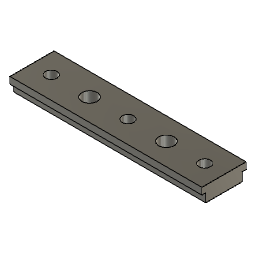
Alu_M6_M8_T-Track_Sliding_nut_T_100mm_holes_int (Autodesk Fusion 360 design; units mm, degrees)
Autodesk Fusion 360 part; units mm, degrees
sketch "Sketch1" plane through (0, 0, 0) normal (1, 0, 0) x (0, 1, 0)
  line L0 (0, 0) -> (9.5, 0)
  line L1 (0, 0) -> (0, 8) construction
  line L2 (0, 8) -> (11.5, 8)
  line L3 (11.5, 8) -> (11.5, 4.5)
  line L4 (11.5, 4.5) -> (9.5, 4.5)
  line L5 (9.5, 4.5) -> (9.5, 0)
  line L6 (-9.5, 4.5) -> (-9.5, 0)
  line L7 (-11.5, 8) -> (-11.5, 4.5)
  line L8 (0, 0) -> (-9.5, 0)
  line L9 (0, 8) -> (-11.5, 8)
  line L10 (-11.5, 4.5) -> (-9.5, 4.5)
  dimension "d1" = 9.5
  dimension "d2" = 8
  dimension "d3" = 11.5
  dimension "d4" = 3.5
  constraint coincident L0.start L1.start
  constraint horizontal L0
  constraint perpendicular L0 L1
  constraint perpendicular L1 L2
  constraint perpendicular L2 L3
  constraint perpendicular L3 L4
  constraint perpendicular L0 L5
  constraint symmetric L0.start L1 L8.start
  constraint symmetric L0.end L1 L6.end
  constraint symmetric L2.start L1 L9.start
  constraint symmetric L1 L2.end L7.start
  constraint symmetric L1 L3.end L7.end
  constraint symmetric L1 L4.end L6.start
  measures "d1" distance of L0.start L0.end
  measures "d2" distance of L0.start L1.end
  measures "d3" distance of L1.end L2.end
  measures "d4" distance of L2.end L3.end
extrude "Extrude1" add sketch "Sketch1" along normal mid plane 100
sketch "Sketch2" plane through (0, 0, 8) normal (0, 0, 1) x (-1, 0, 0)
  line L0 (50, 11.5) -> (-50, 11.5)
  line L1 (-50, 11.5) -> (-50, -11.5)
  line L2 (-50, -11.5) -> (50, -11.5)
  line L3 (50, -11.5) -> (50, 11.5)
  line L4 (50, 0) -> (40, 0) construction
  circle A0 centre (40, 0) radius 3
  line L5 (40, 0) -> (20, 0) construction
  circle A1 centre (20, 0) radius 4
  dimension "d11" = 10
  dimension "d12" = 6
  dimension "d13" = 20
  dimension "d14" = 8
  constraint horizontal L4
  constraint coincident L4.end A0.centre
  constraint parallel L4 L5
  constraint coincident L5.end A1.centre
  measures "d11" distance of L4.start L4.end
  measures "d12" diameter of A0
  measures "d13" distance of L4.end L5.end
  measures "d14" diameter of A1
extrude "Extrude2" cut sketch "Sketch2" against normal up to surface (8 mm away) contours A0 | A1
pattern_linear "R-Pattern1" count 5 spacing 40 along (1, 0, 0) of "Extrude2"
equation "d1 = ( 19 / 2 ) * 1 mm"
equation "d3 = ( 23 / 2 ) * 1 mm"
equation "Alu_M6_M8_T_track_length_slider = 100 mm"
equation "d6 = Alu_M6_M8_T_track_length_slider / 2"
